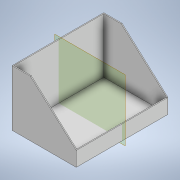
# Autodesk Inventor part: bois
Saved by Autodesk Inventor 2022 (Build 260153000, 153)
## iProperties
Created: 2022-08-02
Part Number: bois
Material: Generic
Document SubType Name: Modeling
Designer: thoma
Density: 1 g/cm^3
Appearance: Default
Author: thoma
Autodesk Inventor part; units mm, degrees
ref_plane "YZ Plane" through (0, 0, 0) normal (1, 0, 0) x (0, 1, 0)
ref_plane "XZ Plane" through (0, 0, 0) normal (0, 1, 0) x (-1, 0, 0)
ref_plane "XY Plane" through (0, 0, 0) normal (0, 0, 1) x (1, 0, 0)
sketch "Sketch2" plane through (0, 0, 0) normal (0, 1, 0) x (-1, 0, 0)
  line L0 (0, 0) -> (700, 0)
  line L1 (700, 0) -> (700, -1000)
  line L2 (700, -1000) -> (0, -1000)
  line L3 (0, -1000) -> (0, 0)
  dimension "d0" = 700
  dimension "d1" = 1000
  constraints: 8 end point, 2 parallel, 1 horizontal, 1 perpendicular
  measures "d0" distance of L0.start L0.end
  measures "d1" distance of L2.end L0.start
extrude "Extrusion1" add sketch "Sketch2" along normal blind 10
sketch "Sketch3" plane through (-700, 0, 0) normal (0, 0, 1) x (1, 0, 0)
  line L0 (700, 10) -> (0, 10) projected
  line L1 (0, 10) -> (0, 610)
  line L2 (0, 610) -> (200, 610)
  line L3 (200, 610) -> (700, 160)
  line L4 (700, 160) -> (700, 10)
  line L5 (0, 10) -> (700, 10)
  line L6 (700, 160) -> (0, 160) construction
  point P0 (700, 0)
  dimension "d4" = 600
  dimension "d5" = 200
  dimension "d6" = 150
  dimension "d13" = 700
  dimension "d14" = 41.987
  constraints: 12 end point, 2 perpendicular, 2 vertical, 1 collinear, 1 point on line
  measures "d4" distance of L0.end L1.end
  measures "d5" distance of L1.end L2.end
  measures "d6" distance of L3.end L0.start
  measures "d13" distance of L0.start L0.end
  measures "d14" angle of L3 L6
extrude "Extrusion2" add sketch "Sketch3" against normal blind 10
ref_plane "Work Plane1" through (0, 0, -500) normal (0, 0, -1) x (-1, 0, 0)
mirror "Mirror1" about plane through (0, 0, -500) normal (0, 0, -1) of "Extrusion2"
sketch "Sketch4" plane through (0, 0, 0) normal (1, 0, 0) x (0, 0, -1)
  line L0 (990, 10) -> (10, 10) projected
  line L1 (1000, 160) -> (990, 160) projected
  line L2 (10, 10) -> (990, 10)
  line L3 (990, 10) -> (990, 160)
  line L4 (990, 160) -> (10, 160)
  line L5 (10, 160) -> (10, 10)
  point P0 (0, 0)
  constraints: 8 end point, 2 parallel, 1 horizontal, 1 perpendicular
extrude "Extrusion3" add sketch "Sketch4" against normal blind 10
sketch "Sketch5" plane through (-700, 0, -1000) normal (-1, 0, 0) x (0, 0, 1)
  line L0 (990, 10) -> (10, 10) projected
  line L1 (990, 10) -> (990, 610) projected
  line L2 (10, 10) -> (990, 10)
  line L3 (990, 10) -> (990, 610)
  line L4 (990, 610) -> (10, 610)
  line L5 (10, 610) -> (10, 10)
  point P0 (1000, 0)
  constraints: 8 end point, 2 parallel, 1 horizontal, 1 perpendicular
extrude "Extrusion4" add sketch "Sketch5" against normal blind 10
body "Solid1"
